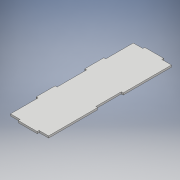
# Autodesk Inventor part: sampingkanan
Saved by Autodesk Inventor 2017 (Build 210142000, 142)
## iProperties
Created: 2017-01-06
Part Number: sampingkanan
Material: Generic
Document SubType Name: Modeling
Designer: Ghesa Bhakti
Density: 1 g/cm^3
Appearance: Default
Author: Ghesa Bhakti
Autodesk Inventor part; units mm, degrees
ref_plane "YZ Plane" through (0, 0, 0) normal (1, 0, 0) x (0, 1, 0)
ref_plane "XZ Plane" through (0, 0, 0) normal (0, 1, 0) x (-1, 0, 0)
ref_plane "XY Plane" through (0, 0, 0) normal (0, 0, 1) x (1, 0, 0)
sketch "Sketch1" plane through (0, 0, 0) normal (0, 0, 1) x (1, 0, 0)
  line L0 (15.0759, 200.5616) -> (15.0759, 197.5616)
  line L1 (45.0759, 197.5616) -> (45.0759, 200.5616)
  line L2 (45.0759, 200.5616) -> (15.0759, 200.5616)
  line L3 (60.0759, 197.5616) -> (45.0759, 197.5616)
  line L4 (15.0759, 197.5616) -> (0.0759, 197.5616)
  line L5 (57.0759, 81.5616) -> (60, 81.5616)
  line L6 (0.0759, 77.6616) -> (-2.9241, 77.6616)
  line L7 (-2.9241, 77.6616) -> (-2.9241, 47.8616)
  line L8 (-2.9241, 47.8616) -> (0.0759, 47.8616)
  line L9 (60, 4.5616) -> (60, 81.5616)
  line L10 (0.0759, 47.8616) -> (0.0759, 4.5616)
  line L11 (0.0759, 4.5616) -> (15.0759, 4.5616)
  line L12 (60.0757, 4.4159) -> (60, 4.5616)
  line L13 (45.0759, 4.4159) -> (60.0757, 4.4159)
  line L14 (45.0759, 4.4159) -> (45.0759, 1.4159)
  line L15 (45.0759, 1.4159) -> (15.0759, 1.5616)
  line L16 (15.0759, 1.5616) -> (15.0759, 4.5616)
  line L17 (0.0759, 197.5616) -> (0.0759, 154.2616)
  line L18 (0.0759, 154.2616) -> (-2.9241, 154.2616)
  line L19 (60.0759, 121.5616) -> (57.0759, 121.5616)
  line L20 (60.0759, 121.5616) -> (60.0759, 197.5616)
  line L21 (57.0759, 121.5616) -> (57.0759, 81.5616)
  line L22 (-2.9241, 124.2616) -> (0.0759, 124.2616)
  line L23 (-2.9241, 154.2616) -> (-2.9241, 124.2616)
  line L24 (0.0759, 124.2616) -> (0.0759, 77.6616)
  point P0 (0, 0)
  dimension "d25" = 193
  dimension "d26" = 60
  dimension "d27" = 3
  dimension "d28" = 30
  dimension "d29" = 15
  dimension "d30" = 3
  dimension "d31" = 3
  dimension "d32" = 15
  dimension "d33" = 3
  dimension "d34" = 3
  dimension "d35" = 3
  dimension "d36" = 3
  dimension "d37" = 15
  dimension "d38" = 40
  dimension "d39" = 3
  dimension "d41" = 77
  dimension "d43" = 3
  dimension "d44" = 76
  dimension "d45" = 199.1457
  dimension "d46" = 43.3
  dimension "d47" = 46.6
  dimension "d48" = 43.3
  dimension "d49" = 30
  dimension "d50" = 29.8
  constraints: 50 end point, 9 parallel, 5 horizontal, 3 perpendicular, 2 vertical, 1 point on line
  measures "d25" distance of L4.end L10.end
  measures "d26" distance of L10.end L12.start
  measures "d27" distance of L3.end L1.end
  measures "d28" distance of L1.end L0.start
  measures "d29" distance of L0.end L4.end
  measures "d30" distance of L17.end L18.end
  measures "d31" distance of L6.start L6.end
  measures "d32" distance of L3.start L3.end
  measures "d33" distance of L7.end L8.end
  measures "d34" distance of L22.start L22.end
  measures "d35" distance of L13.start L14.end
  measures "d36" distance of L15.end L11.end
  measures "d37" distance of L10.end L11.end
  measures "d38" distance of L19.end L5.start
  measures "d39" distance of L20.start L19.end
  measures "d41" distance of L9.start L5.end
  measures "d43" distance of L0.start L0.end
  measures "d44" distance of L20.start L3.start
  measures "d45" distance of L14.end L1.end
  measures "d46" distance of L4.end L17.end
  measures "d47" distance of L22.end L6.start
  measures "d48" distance of L8.end L10.end
  measures "d49" distance of L18.end L22.start
  measures "d50" distance of L6.end L7.end
extrude "Extrusion1" add sketch "Sketch1" along normal blind 3
body "Solid1"
